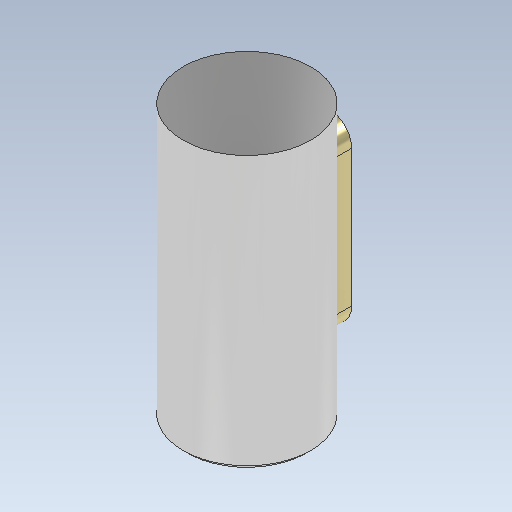
# Autodesk Inventor part: inputshaft nmrv50
Saved by Autodesk Inventor 2020 (Build 240168000, 168)
## iProperties
Created: 2020-07-31
Part Number: inputshaft nmrv50
Material: Generic
Document SubType Name: Modeling
Designer: Vikki
Density: 1 g/cm^3
Appearance: Chrome - Polished
Mass: 4.58941 g
Surface Area: 18.7189 cm^2
Volume: 4.58941 cm^3
Author: Vikki
Autodesk Inventor part; units mm, degrees
ref_plane "YZ Plane" through (0, 0, 0) normal (1, 0, 0) x (0, 1, 0)
ref_plane "XZ Plane" through (0, 0, 0) normal (0, 1, 0) x (-1, 0, 0)
sketch "Sketch1" plane through (0, 0, 0) normal (0, 1, 0) x (-1, 0, 0)
  circle A0 centre (0, 0) radius 7
  dimension "d0" = 14
  constraints: 1 centre point, 1 coincident
  measures "d0" diameter of A0
extrude "Extrusion1" add sketch "Sketch1" along normal blind 30
sketch "Sketch2" plane through (0, 0, 0) normal (0, -1, 0) x (1, 0, 0)
  point P0 (0, 0)
ref_plane "Work Plane1" through (0, 0, -7) normal (0, 0, 1) x (1, 0, 0)
sketch "Sketch3" plane through (0, 0, -7) normal (0, 0, 1) x (1, 0, 0)
  line L0 (0, 5) -> (0, 5)
  line L1 (-2.5, 7.5) -> (-2.5, 22.5)
  line L2 (0, 25) -> (0, 25)
  line L3 (2.5, 22.5) -> (2.5, 7.5)
  line L4 (7, 0) -> (-7, 0) projected
  arc A0 (0, 5) -> (2.5, 7.5) centre (0, 7.5) ccw
  arc A1 (-2.5, 7.5) -> (0, 5) centre (0, 7.5) ccw
  arc A2 (0, 25) -> (-2.5, 22.5) centre (0, 22.5) ccw
  arc A3 (2.5, 22.5) -> (0, 25) centre (0, 22.5) ccw
  point P0 (0, 0)
  point P1 (2.5, 5)
  point P2 (2.5, 25)
  point P3 (0, 5)
  point P4 (0, 25)
  dimension "d3" = 5
  dimension "d4" = 20
  dimension "d5" = 5
  dimension "d6" = 2.5
  dimension "d7" = 2.5
  constraints: 8 end point, 8 point on circle, 8 tangent, 4 centre point, 4 point on line, 3 equal radius, 2 parallel, 1 horizontal, 1 perpendicular
  measures "d3" distance between parallel lines of L0 L4
  measures "d4" distance of point (2.5, 25) point (2.5, 5)
  measures "d5" distance between parallel lines of L1 L3
  measures "d6" horizontal distance of point (0, 0) point (2.5, 5)
  measures "d7" radius of A0
extrude "Extrusion2" add sketch "Sketch3" along normal blind 1 and the other way blind 2
sketch "Sketch4" plane through (0, 0, 0) normal (0, -1, 0) x (1, 0, 0)
  circle A0 centre (0, 0) radius 3
  dimension "d12" = 6
  constraints: 1 centre point, 1 coincident
  measures "d12" diameter of A0
extrude "Extrusion3" cut sketch "Sketch4" against normal blind 8
chamfer "Chamfer1" distance 0.5 angle 45 1 edges at (7, 0, 0)
thread "Thread1" size "M6x1" class "6H" standard "ANSI Metric M Profile" length 60
body "Solid1"
